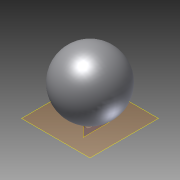
# Autodesk Inventor part: Ball
Saved by Autodesk Inventor 2012 SP2 (Build 160219200, 219)
## iProperties
Created: 2014-02-08
Part Number: Ball
Material: Default
Document SubType Name: Modeling
Designer: 1
Density: 1 g/cm^3
Author: 1
Autodesk Inventor part; units mm, degrees
ref_plane "YZ Plane" through (0, 0, 0) normal (1, 0, 0) x (0, 1, 0)
ref_plane "XY Plane" through (0, 0, 0) normal (0, 0, 1) x (1, 0, 0)
sketch "Sketch1" plane through (0, 0, 0) normal (0, 0, 1) x (1, 0, 0)
  circle A0 centre (-13.65, 389.8638) radius 26.3731
  line L0 (-12.9219, 135.373) -> (-12.9219, 344.0738)
  line L1 (-14.3781, 135.373) -> (-14.3781, 344.0738)
  line L2 (-14.3781, 344.0738) -> (-12.9219, 344.0738)
  line L3 (-13.65, 344.0738) -> (-13.65, 443.1033)
  line L4 (-13.65, 363.4908) -> (-13.65, 416.2369)
  point P0 (0, 0)
  constraints: 10 end point, 3 point on line, 2 perpendicular, 2 point on circle, 2 vertical, 1 centre point, 1 midpoint, 4 other
revolve "Revolution1" add sketch "Sketch1" angle 360 about axis through (-13.65, 344.0738, 0) along (0, 1, 0) picked at (-15.7538, 398.3994) contours L3 A0
ref_plane "Work Plane1" through (-13.65, 363.4908, 0) normal (0, 1, 0) x (-1, 0, 0)
sketch "Sketch2" plane through (-13.65, 363.4908, 0) normal (0, 1, 0) x (-1, 0, 0)
  circle A0 centre (0.0061, -5.1267) radius 1.2823
  line L0 (-16.2825, 0) -> (16.6651, 0)
  circle A1 centre (0.0061, 5.1267) radius 1.2823
  point P0 (-13.65, 0)
  constraints: 2 centre point, 2 end point, 1 horizontal, 1 symmetric about line, 1 other
ref_plane "Work Plane2" through (-13.6561, 363.4908, -5.1267) normal (-1, 0, 0) x (0, -1, 0)
sketch "Sketch3" plane through (-13.6561, 363.4908, -5.1267) normal (-1, 0, 0) x (0, -1, 0)
  line L0 (0, 10.2534) -> (-8.6144, 10.2534)
  line L1 (0, 0) -> (-6.0863, 0)
  line L2 (0, -31.7956) -> (0, 42.0491) projected
  line L3 (0, 1.2823) -> (0, -1.2823) projected
  arc A0 (0, 0) -> (0, 10.2534) centre (0, 5.1267) ccw
  line L4 (-8.6144, 10.2534) -> (-6.0863, 0)
  point P0 (363.4908, 5.1267)
  dimension "d1" = 103.851
  dimension "d2" = 360.0583
  constraints: 6 end point, 2 horizontal, 2 point on circle, 2 point on line, 1 centre point, 1 tangent
  measures "d1" angle of L4 L0
  measures "d2" distance from line of point (363.491, 5.127) L4
sweep "Sweep1" add profiles "Sketch2" path "Sketch3" path curves A0 L0 L4 L1 contours A1
body "Solid1"
